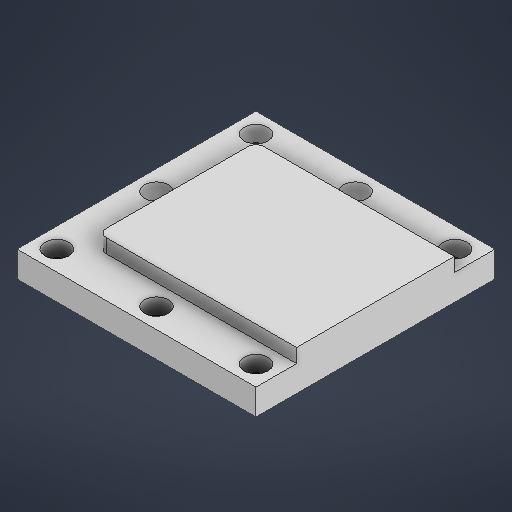
# Autodesk Inventor part: Flex Circuit Clamp Base V1
Saved by Autodesk Inventor 2026.2 (Build 302298010, 298A)
## iProperties
Created: 2026-05-04
Part Number: Flex Circuit Clamp Base V1
Material: Generic
Document SubType Name: Modeling
Designer: cfang
Density: 1 g/cm^3
Appearance: Default
Author: cfang
Autodesk Inventor part; units mm, degrees
ref_plane "YZ Plane" through (0, 0, 0) normal (1, 0, 0) x (0, 1, 0)
ref_plane "XZ Plane" through (0, 0, 0) normal (0, 1, 0) x (-1, 0, 0)
ref_plane "XY Plane" through (0, 0, 0) normal (0, 0, 1) x (1, 0, 0)
sketch "Sketch1" plane through (0, 0, 0) normal (0, 1, 0) x (-1, 0, 0)
  line L0 (-15, -15) -> (15, -15)
  line L1 (15, -15) -> (15, 15)
  line L2 (15, 15) -> (-15, 15)
  line L3 (-15, 15) -> (-15, -15)
  line L4 (-15, -15) -> (15, 15) construction
  line L5 (15, -15) -> (-15, 15) construction
  point P0 (0, 0)
  dimension "d0" = 30
  dimension "d1" = 30
  constraints: 12 end point, 2 midpoint, 2 parallel, 1 horizontal, 1 perpendicular
  measures "d0" distance of L0.end L1.end
  measures "d1" distance of L1.end L2.end
extrude "Extrusion1" add sketch "Sketch1" along normal blind 5
sketch "Sketch2" plane through (0, 5, 0) normal (0, 1, 0) x (1, 0, 0)
  line L0 (-15, -15) -> (15, -15) projected
  line L1 (-15, 15) -> (-15, -15) projected
  line L2 (15, 15) -> (-15, 15) projected
  line L3 (15, -15) -> (15, 15) projected
  line L4 (-15, -15) -> (15, -15)
  line L5 (15, -15) -> (15, -9.9)
  line L6 (15, -9.9) -> (-8.9, -9.9)
  line L7 (-15, -9.9) -> (-15, -15)
  line L8 (-15, -15) -> (-9.9, -15)
  line L9 (-9.9, -8.9) -> (-9.9, 8.9)
  line L10 (-9.9, 15) -> (-15, 15)
  line L11 (-15, 15) -> (-15, -15)
  line L12 (15, 15) -> (-9.9, 15)
  line L13 (-9.9, 15) -> (-9.9, 9.9)
  line L14 (-8.9, 9.9) -> (15, 9.9)
  line L15 (15, 9.9) -> (15, 15)
  arc A0 (-9.9, -8.9) -> (-8.9, -9.9) centre (-8.9, -8.9) ccw
  arc A1 (-8.9, 9.9) -> (-9.9, 8.9) centre (-8.9, 8.9) ccw
  point P0 (0, 0)
  dimension "d4" = 5.1
  dimension "d5" = 5.1
  dimension "d6" = 5.1
  dimension "d7" = 1
  constraints: 24 end point, 7 point on line, 6 parallel, 4 point on circle, 4 tangent, 3 horizontal, 3 perpendicular, 2 centre point, 1 equal radius
  measures "d4" distance between parallel lines of L0 L6
  measures "d5" distance between parallel lines of L14 L2
  measures "d6" distance between parallel lines of L1 L9
  measures "d7" radius of A0
extrude "Extrusion2" cut sketch "Sketch2" against normal blind 1.75 contours L1 L2 L3 L14 A1 L9 A0 L6 L0
sketch "Sketch3" plane through (0, 3.25, 0) normal (0, 1, 0) x (1, 0, 0)
  line L0 (-9.9, 8.9) -> (-9.9, -8.9) projected
  line L1 (15, -15) -> (-15, -15) projected
  line L2 (-15, 15) -> (15, 15) projected
  point P0 (0, 0)
  point P1 (-12.5, -12.5)
  point P2 (12.5, -12.5)
  point P3 (-12.5, 12.5)
  point P4 (12.5, 12.5)
  point P5 (-9.9, 0)
  point P6 (0, -15)
  point P7 (0, -12.5)
  point P8 (-12.5, 0)
  point P9 (0, 12.5)
  point P10 (-9.9, 0)
  point P11 (0, -15)
  point P12 (0, 15)
  dimension "d10" = 25
  dimension "d11" = 25
  dimension "d12" = 12.5
  dimension "d13" = 12.5
  constraints: 5 horizontal alignment, 5 midpoint, 5 vertical alignment
  measures "d10" distance of point (12.5, -12.5) point (-12.5, -12.5)
  measures "d11" distance of point (-12.5, 12.5) point (-12.5, -12.5)
  measures "d12" vertical distance of point (-12.5, -12.5) point (-9.9, 0)
  measures "d13" horizontal distance of point (-12.5, -12.5) point (0, -15)
hole "Hole1" at (-12.5, 3.25, 12.5) at (12.5, 3.25, 12.5) at (-12.5, 3.25, -12.5) at (12.5, 3.25, -12.5) at (0, 3.25, 12.5) at (0, 3.25, -12.5) at (-12.5, 3.25, 0) direction (0, -1, 0) diameter 3 depth 2
hole "Hole2" at (-12.5, 3.25, 0) at (-12.5, 3.25, 12.5) at (0, 3.25, 12.5) at (12.5, 3.25, 12.5) at (12.5, 3.25, -12.5) at (0, 3.25, -12.5) at (-12.5, 3.25, -12.5) direction (0, -1, 0) diameter 2.2 end through all
equation "\"d5\" = d4"
equation "\"d6\" = d4"
equation "\"d12\" = 0.5 * d11"
equation "\"d13\" = 0.5 * d10"
body "Solid1"
